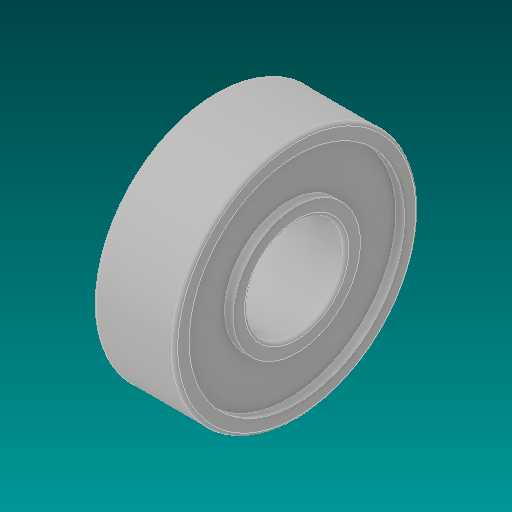
# Autodesk Inventor part: B696ZZ
Saved by Autodesk Inventor 2020 (Build 240168000, 168)
## iProperties
Created: 2022-11-16
Part Number: B696ZZ
Material: Generic
Catalog Web Link: www.cadenas.de
Description: B6 _ _ ZZ, B6 _ _ AZZ, SB6 _ _ ZZ, SB6 _ _ AZZ, BR _ _ ZZ, SBR _ _ ZZ-Small Ball Bearings - Double Shield Type
Vendor: MISUMI
Document SubType Name: Modeling
Designer: psAdmin
Manufacturer: MISUMI
Mass: 0.647818 g
Surface Area: 6.84496 cm^2
Volume: 0.647818 cm^3
Density: 1 g/cm^3
Appearance: PSOLRGB-175-175-175
Category: PARTsolutions
Company: MISUMI
PSOL_IDENT_0: {$CADENAS_DATA/23d-libs/misumi/metric/12_bearing_holders/sb685zz.prj},219 {VTYP=3D},{NB=B696ZZ},{LIN
PSOL_IDENT_1: A=B696ZZ},{NN=B6 _ _ ZZ, B6 _ _ AZZ, SB6 _ _ ZZ, SB6 _ _ AZZ, BR _ _ ZZ, SBR _ _ ZZ},{DATE=30.06.202
PSOL_IDENT_2: 1 12:59:24},{GEOMDATE=23.07.2013 00:00:00},{VERSION=},{LINEID=120},{WBVAR=MAT},{WBNUMERIC=}  {NB=B69
PSOL_IDENT_3: 6ZZ},{LINA=B696ZZ},{KT=DUMMY},{PN=B696ZZ},{MAT=},{BN=696ZZ},{DD=6.0},{A=3.9530},{BB=0.900},{C=0.900}
PSOL_IDENT_4: ,{D=15},{B=5.0},{RR=0.20},{CR=1350},{COR=530},{CRS=1350},{CRSS=1139},{CORS=530},{CORSS=418},{DS=7.60
PSOL_IDENT_5: },{DDHH=13.40},{R=0.20},{MASS=3.8},{X=0},{BN2=B696ZZ}
NB: B696ZZ
NN: B6 _ _ ZZ, B6 _ _ AZZ, SB6 _ _ ZZ, SB6 _ _ AZZ, BR _ _ ZZ, SBR _ _ ZZ
NT: Small Ball Bearings - Double Shield Type
NBSYN: $PN.
LINA: B696ZZ
CATALOG: Misumi
PN: B696ZZ
MAT: 52100 Bearing Steel
BN: 696ZZ
DD: 6
D: 15
B: 5
RR: 0.2
CR: 1350
COR: 530
DS: 7.6
DDHH: 13.4
R: 0.2
MASS: 3.8
X: 0
SUPPLIER: MISUMI
ARTICLENO: B696ZZ
BOMINFO: B696ZZ
CREATOR: CADENAS GmbH
d1: 0.000 mm
Title: B696ZZ
Author: Cadenas PARTsolutions
Comments: Small Ball Bearings - Double Shield Type
Autodesk Inventor part; units mm, degrees
sketch "Sketch_1" plane through (0, 0, 0) normal (0, 0, 1) x (1, 0, 0)
  line L0 (4.8, 0) -> (0.2, 0)
  arc A0 (0, 3.2) -> (0.2, 3) centre (0.2, 3.2) ccw
  line L1 (0.2, 3) -> (4.8, 3)
  arc A1 (4.8, 3) -> (5, 3.2) centre (4.8, 3.2) ccw
  line L2 (5, 3.2) -> (5, 3.9)
  line L3 (5, 3.9) -> (4.4765, 3.9)
  line L4 (4.4765, 3.9) -> (4.4765, 6.6)
  line L5 (4.4765, 6.6) -> (5, 6.6)
  line L6 (5, 6.6) -> (5, 7.3)
  arc A2 (5, 7.3) -> (4.8, 7.5) centre (4.8, 7.3) ccw
  line L7 (4.8, 7.5) -> (0.2, 7.5)
  arc A3 (0.2, 7.5) -> (0, 7.3) centre (0.2, 7.3) ccw
  line L8 (0, 7.3) -> (0, 6.6)
  line L9 (0, 6.6) -> (0.5235, 6.6)
  line L10 (0.5235, 6.6) -> (0.5235, 3.9)
  line L11 (0.5235, 3.9) -> (0, 3.9)
  line L12 (0, 3.9) -> (0, 3.2)
  constraints: 26 end point, 8 point on circle, 4 centre point
revolve "Revolution1" add sketch "Sketch_1" angle 360 about axis through (4.8, 0, 0) along (1, 0, 0)
ref_plane "to_housing_XY" through (0, 0, 0) normal (1, 0, 0) x (0, 0, -1)
ref_plane "to_housing_YZ" through (0, 0, 0) normal (0, 0, -1) x (0, 1, 0)
ref_plane "to_housing_ZX" through (0, 0, 0) normal (0, 1, 0) x (1, 0, 0)
ref_plane "to_housing_center_XY" through (2.5, 0, 0) normal (1, 0, 0) x (0, 0, -1)
ref_plane "to_housing_center_YZ" through (2.5, 0, 0) normal (0, 0, -1) x (0, 1, 0)
ref_plane "to_housing_center_ZX" through (2.5, 0, 0) normal (0, 1, 0) x (1, 0, 0)
body "Solid1"
